Kindersicherung_Schranktueren_Unterteller_M3_v2 (Autodesk Fusion 360 design; units mm, degrees)
Autodesk Fusion 360 part; units mm, degrees
sketch "Sketch1" plane through (0, 0, 0) normal (0, 1, 0) x (1, 0, 0)
  circle A0 centre (0, 0) radius 16.5
  dimension "d1" = 33
  constraint coincident A0.centre origin
  measures "d1" diameter of A0
extrude "Extrude1" add sketch "Sketch1" along normal blind 1.5
sketch "Sketch2" plane through (0, 1.5, 0) normal (0, 1, 0) x (-1, 0, 0)
  circle A0 centre (0, 0) radius 16.5
  circle A1 centre (0, 0) radius 3
  circle A2 centre (0, 0) radius 1.45
  dimension "d4" = 6
  dimension "d5" = 2.9
  constraint coincident A0.centre A1.centre
  measures "d4" diameter of A1
  measures "d5" diameter of A2
extrude "Extrude2" add sketch "Sketch2" along normal blind 7 contours A1
fillet "Fillet1" radius 0.5 3 edges at (-15.3834, 0, 5.9667) (-15.3834, 1.5, 5.9667) (2.797, 8.5, -1.0848)
